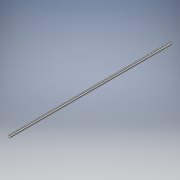
# Autodesk Inventor part: ThunderHex36
Saved by Autodesk Inventor 2018.3 (Build 223284000, 284)
## iProperties
Created: 2019-03-03
Part Number: ThunderHex36
Material: Generic
Document SubType Name: Modeling
Designer: Srinity
Density: 1 g/cm^3
Appearance: Default
Author: Srinity
Autodesk Inventor part; units mm, degrees
ref_plane "YZ Plane" through (0, 0, 0) normal (1, 0, 0) x (0, 1, 0)
ref_plane "XZ Plane" through (0, 0, 0) normal (0, 1, 0) x (-1, 0, 0)
ref_plane "XY Plane" through (0, 0, 0) normal (0, 0, 1) x (1, 0, 0)
sketch "Sketch1" plane through (0, 0, 0) normal (0, 0, 1) x (1, 0, 0)
  arc A0 (-5.109, 4.6004) -> (-6.8651, -0.3684) centre (0, 0) ccw
  line L0 (-4.7654, 5.5726) -> (-3.7516, 5.7612)
  line L1 (2.4434, 6.9133) -> (3.1135, 6.1296)
  line L2 (7.2087, 1.3406) -> (6.8651, 0.3684)
  line L3 (4.7654, -5.5726) -> (3.7516, -5.7612)
  line L4 (-2.4434, -6.9133) -> (-3.1135, -6.1296)
  line L5 (-7.2087, -1.3406) -> (-6.8651, -0.3684)
  arc A1 (-3.7516, 5.7612) -> (-5.109, 4.6004) centre (0, 0) ccw
  arc A2 (1.4295, 6.7247) -> (-3.7516, 5.7612) centre (0, 0) ccw
  arc A3 (3.1135, 6.1296) -> (1.4295, 6.7247) centre (0, 0) ccw
  arc A4 (6.5386, 2.1243) -> (3.1135, 6.1296) centre (0, 0) ccw
  arc A5 (6.8651, 0.3684) -> (6.5386, 2.1243) centre (0, 0) ccw
  arc A6 (5.109, -4.6004) -> (6.8651, 0.3684) centre (0, 0) ccw
  arc A7 (3.7516, -5.7612) -> (5.109, -4.6004) centre (0, 0) ccw
  arc A8 (-1.4295, -6.7247) -> (3.7516, -5.7612) centre (0, 0) ccw
  arc A9 (-3.1135, -6.1296) -> (-1.4295, -6.7247) centre (0, 0) ccw
  arc A10 (-6.5386, -2.1243) -> (-3.1135, -6.1296) centre (0, 0) ccw
  arc A11 (-6.8651, -0.3684) -> (-6.5386, -2.1243) centre (0, 0) ccw
  line L6 (-5.109, 4.6004) -> (-4.7654, 5.5726)
  line L7 (-6.8651, -0.3684) -> (-5.109, 4.6004)
  line L8 (-6.5386, -2.1243) -> (-7.2087, -1.3406)
  line L9 (-3.1135, -6.1296) -> (-6.5386, -2.1243)
  line L10 (-1.4295, -6.7247) -> (-2.4434, -6.9133)
  line L11 (3.7516, -5.7612) -> (-1.4295, -6.7247)
  line L12 (5.109, -4.6004) -> (4.7654, -5.5726)
  line L13 (6.8651, 0.3684) -> (5.109, -4.6004)
  line L14 (6.5386, 2.1243) -> (7.2087, 1.3406)
  line L15 (3.1135, 6.1296) -> (6.5386, 2.1243)
  line L16 (1.4295, 6.7247) -> (2.4434, 6.9133)
  line L17 (-3.7516, 5.7612) -> (1.4295, 6.7247)
  dimension "d0" = 12.7
  dimension "d1" = 13.75
  constraints: 36 end point, 24 point on circle, 12 centre point, 2 coincident, 13 other
  measures "d0" distance between parallel lines of L3 L0
  measures "d1" diameter of A0
extrude "Extrusion1" add sketch "Sketch1" along normal blind 914.4 contours A1 L17 A3 L15 A5 L13 A7 L11 A9 L9 A11 L7
body "Solid1"
